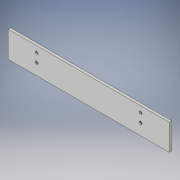
# Autodesk Inventor part: tyl
Saved by Autodesk Inventor 2019 (Build 230136000, 136)
## iProperties
Created: 2019-09-07
Part Number: tyl
Material: Generic
Document SubType Name: Modeling
Designer: Michal
Density: 1 g/cm^3
Appearance: Default
Author: Michal
Autodesk Inventor part; units mm, degrees
ref_plane "YZ Plane" through (0, 0, 0) normal (1, 0, 0) x (0, 1, 0)
ref_plane "XZ Plane" through (0, 0, 0) normal (0, 1, 0) x (-1, 0, 0)
ref_plane "XY Plane" through (0, 0, 0) normal (0, 0, 1) x (1, 0, 0)
sketch "Sketch1" plane through (0, 0, 0) normal (0, 0, 1) x (1, 0, 0)
  line L0 (0, 0) -> (-186, 0)
  line L1 (-186, 0) -> (-186, 30)
  line L2 (-186, 30) -> (0, 30)
  line L3 (0, 30) -> (0, 0)
  dimension "d0" = 186
  dimension "d1" = 30
  constraints: 8 end point, 2 parallel, 1 horizontal, 1 perpendicular
  measures "d0" distance of L1.end L2.end
  measures "d1" distance of L0.end L1.end
extrude "Extrusion1" add sketch "Sketch1" along normal blind 3
sketch "Sketch2" plane through (0, 0, 0) normal (0, 0, -1) x (-1, 0, 0)
  line L0 (0, 0) -> (186, 0) projected
  line L1 (0, 0) -> (33, 0)
  line L2 (33, 0) -> (33, 13)
  line L3 (33, 13) -> (0, 13)
  line L4 (0, 13) -> (0, 0)
  line L5 (0, 30) -> (186, 30) projected
  line L6 (0, 30) -> (32.9946, 30)
  line L7 (32.9946, 30) -> (32.9946, 23)
  line L8 (32.9946, 23) -> (0, 23)
  line L9 (0, 23) -> (0, 30)
  line L10 (186, 0) -> (153, 0)
  line L11 (153, 0) -> (153, 13)
  line L12 (153, 13) -> (186, 13)
  line L13 (186, 13) -> (186, 0)
  line L14 (186, 30) -> (153, 30)
  line L15 (153, 30) -> (153, 23)
  line L16 (153, 23) -> (186, 23)
  line L17 (186, 23) -> (186, 30)
  dimension "d16" = 33
  dimension "d17" = 13
  dimension "d18" = 32.9946
  dimension "d19" = 7
  dimension "d20" = 33
  constraints: 32 end point, 8 parallel, 4 horizontal, 4 perpendicular, 2 point on line
  measures "d16" distance of L3.end L2.end
  measures "d17" distance of L2.end L1.end
  measures "d18" distance of L7.end L8.end
  measures "d19" distance of L6.end L7.end
  measures "d20" distance of L11.end L12.end
hole "Hole1" at (-32.9946, 23, 0) at (-33, 13, 0) at (-153, 23, 0) at (-153, 13, 0) direction (0, 0, 1) diameter 3.4 end through all countersink diameter 6.9 countersink angle 89.954 clearance for "Countersunk Flat Head Screw ISO 2009/7046" size "M3" standard "ISO"
body "Solid1"
